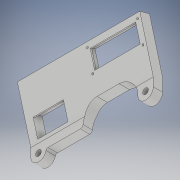
# Autodesk Inventor part: dash
Saved by Autodesk Inventor 2019 (Build 230136000, 136)
## iProperties
Created: 2019-09-21
Part Number: dash
Material: Generic
Document SubType Name: Modeling
Designer: steve
Density: 1 g/cm^3
Appearance: Default
Author: steve
Autodesk Inventor part; units mm, degrees
ref_plane "YZ Plane" through (0, 0, 0) normal (1, 0, 0) x (0, 1, 0)
ref_plane "XZ Plane" through (0, 0, 0) normal (0, 1, 0) x (-1, 0, 0)
ref_plane "XY Plane" through (0, 0, 0) normal (0, 0, 1) x (1, 0, 0)
sketch "Sketch1" plane through (0, 0, 0) normal (0, 1, 0) x (-1, 0, 0)
  line L0 (0, 0) -> (0, -18.7068)
  line L1 (0, -18.7068) -> (19.6073, -91.8823)
  line L2 (0, 0) -> (0, 11.24)
  line L3 (0, 11.24) -> (14, 11.24)
  line L4 (14, 11.24) -> (14, -13)
  line L5 (14, -13) -> (34.0962, -88)
  line L6 (34.0962, -88) -> (19.6073, -91.8823)
  dimension "d1" = 14
  dimension "d2" = 11.24
  dimension "d4" = 15
  dimension "d13" = 15
  dimension "d14" = 13
  dimension "d35" = 88
  constraints: 14 end point, 3 perpendicular, 2 vertical, 1 parallel
  measures "d1" distance of L2.end L3.end
  measures "d2" distance of L0.start L2.end
  measures "d4" angle of L0 L1
  measures "d13" distance of L5.end L1.end
  measures "d14" vertical distance of L4.end L0.start
  measures "d35" vertical distance of L5.end L0.start
extrude "Extrusion1" add sketch "Sketch1" along normal blind 183
sketch "Sketch2" plane through (-14, 0, -13) normal (-1, 0, 0) x (0, 0, 1)
  line L0 (0, 183) -> (24.24, 183) projected
  circle A0 centre (12.74, 171.5) radius 4.25
  circle A1 centre (12.74, 11.5) radius 4.25
  line L1 (24.24, 0) -> (24.24, 183) projected
  line L2 (0, 0) -> (24.24, 0) projected
  arc A2 (12.74, 0) -> (15.1193, 22.7512) centre (12.74, 11.5) ccw
  arc A3 (12.2608, 160.01) -> (12.74, 183) centre (12.74, 171.5) ccw
  line L3 (-13.26, 102.4155) -> (-13.26, 135.5313)
  arc A4 (12.2608, 160.01) -> (-13.26, 135.5313) centre (11.24, 135.5313) ccw
  circle A5 centre (20.1015, 118.5) radius 28 construction
  line L4 (12.74, 25.6863) -> (12.74, 74.0254)
  arc A6 (12.74, 25.6863) -> (15.1193, 22.7512) centre (15.74, 25.6863) ccw
  arc A7 (-13.26, 102.4155) -> (9.0909, 78.01) centre (11.24, 102.4155) ccw
  arc A8 (12.74, 74.0254) -> (9.0909, 78.01) centre (8.74, 74.0254) ccw
  line L5 (24.24, 0) -> (24.24, 183) projected
  line L6 (12.74, 0) -> (24.24, 0)
  line L7 (24.24, 11.5) -> (24.24, 171.5)
  line L8 (24.24, 183) -> (12.74, 183)
  line L9 (24.24, 11.5) -> (24.24, 0)
  line L10 (24.24, 171.5) -> (24.24, 183)
  point P0 (13, 0)
  point P1 (12.74, 23)
  point P2 (12.74, 77.9615)
  dimension "d17" = 160
  dimension "d18" = 183
  dimension "d19" = 11.5
  dimension "d20" = 11.5
  dimension "d21" = 11.5
  dimension "d22" = 26
  dimension "d23" = 56
  dimension "d24" = 53
  dimension "d25" = 3
  dimension "d26" = 0
  dimension "d27" = 24.5
  dimension "d28" = 4
  dimension "d30" = 82
  dimension "d31" = 8.5
  dimension "d32" = 4.1385
  constraints: 16 point on circle, 14 end point, 11 tangent, 9 centre point, 4 collinear, 4 point on line, 2 coincident, 2 equal radius, 2 vertical, 1 perpendicular
  measures "d17" distance of A0.centre A1.centre
  measures "d18" distance of L1.start L0.end
  measures "d19" distance from line of L2 A1.centre
  measures "d20" distance from line of L1 A1.centre
  measures "d21" distance from line of L1 A0.centre
  measures "d22" distance from line of A1.centre L3
  measures "d23" diameter of A5
  measures "d24" vertical distance of A0.centre A5.centre
  measures "d25" radius of A6
  measures "d26" distance from line of A1.centre L4
  measures "d27" radius of A4
  measures "d28" radius of A8
  measures "d30" vertical distance of A3.start A7.end
  measures "d31" diameter of A1
  measures "d32" distance from line of A5.centre L1
extrude "Extrusion2" cut sketch "Sketch2" along normal through all both and the other way through all
sketch "Sketch3" plane through (-34.0962, 0, -88) normal (-0.9659258, 0, 0.258819) x (0.258819, 0, 0.9659258)
  line L0 (46.9516, 11.5) -> (72.9516, 11.5)
  line L1 (72.9516, 11.5) -> (72.9516, 56.75)
  line L2 (72.9516, 56.75) -> (46.9516, 56.75)
  line L3 (46.9516, 56.75) -> (46.9516, 11.5)
  ellipse E0 centre (89.9516, 11.5) end of major axis (89.9516, 23) minor radius 11.1081 (89.9516, 0) -> (92.2498, 22.7512) ccw projected
  line L4 (8.9516, 106.5) -> (34.9516, 106.5)
  line L5 (34.9516, 106.5) -> (34.9516, 174.5)
  line L6 (34.9516, 174.5) -> (8.9516, 174.5)
  line L7 (8.9516, 174.5) -> (8.9516, 106.5)
  circle A0 centre (6.4516, 103) radius 1.4
  circle A1 centre (37.4516, 103) radius 1.4
  circle A2 centre (37.4516, 178) radius 1.4
  circle A3 centre (6.4516, 178) radius 1.4
  line L8 (6.4516, 103) -> (37.4516, 103) construction
  line L9 (37.4516, 103) -> (37.4516, 178) construction
  line L10 (37.4516, 178) -> (6.4516, 178) construction
  line L11 (6.4516, 178) -> (6.4516, 103) construction
  point P0 (93.8262, 0)
  dimension "d36" = 45.25
  dimension "d37" = 26
  dimension "d38" = 17
  dimension "d39" = 0
  dimension "d46" = 26
  dimension "d47" = 31
  dimension "d48" = 75
  dimension "d49" = 3.5
  dimension "d50" = 68
  dimension "d51" = 2.5
  dimension "d52" = 55
  dimension "d53" = 95
  dimension "d54" = 2.8
  constraints: 24 end point, 6 parallel, 4 centre point, 3 equal radius, 3 horizontal, 3 perpendicular, 2 coincident, 1 other
  measures "d36" distance of L2.end L0.start
  measures "d37" distance of L1.end L2.end
  measures "d38" distance from line of point (89.952, 11.5) L1
  measures "d39" distance from line of point (89.952, 11.5) L0
  measures "d46" distance of L4.start L4.end
  measures "d47" distance of L9.end L10.end
  measures "d48" distance of L10.end L8.start
  measures "d49" distance between parallel lines of L8 L4
  measures "d50" distance of L6.end L4.start
  measures "d51" distance between parallel lines of L11 L7
  measures "d52" horizontal distance of point (89.952, 11.5) L4.end
  measures "d53" vertical distance of point (89.952, 11.5) L4.end
  measures "d54" diameter of A0
extrude "top" cut sketch "Sketch3" against normal blind 183
sketch "Sketch4" plane through (-19.6073, 0, -91.8823) normal (0.9659258, 0, -0.258819) x (-0.258819, 0, -0.9659258)
  line L0 (-46.9516, 56.75) -> (-46.9516, 11.5) projected
  line L1 (-72.9516, 11.5) -> (-72.9516, 56.75) projected
  line L2 (-42.9516, 56.75) -> (-76.9516, 56.75)
  line L3 (-76.9516, 56.75) -> (-76.9516, 11.5)
  line L4 (-76.9516, 11.5) -> (-42.9516, 11.5)
  line L5 (-42.9516, 11.5) -> (-42.9516, 56.75)
  line L6 (-72.9516, 56.75) -> (-46.9516, 56.75) projected
  line L7 (-46.9516, 11.5) -> (-72.9516, 11.5) projected
  line L8 (-3.9516, 180.5) -> (-39.9516, 180.5)
  line L9 (-39.9516, 180.5) -> (-39.9516, 100.5)
  line L10 (-39.9516, 100.5) -> (-3.9516, 100.5)
  line L11 (-3.9516, 100.5) -> (-3.9516, 180.5)
  circle A0 centre (-6.4516, 103) radius 1.4 projected
  circle A1 centre (-6.4516, 178) radius 1.4 projected
  circle A2 centre (-37.4516, 178) radius 1.4 projected
  point P0 (-93.8262, 0)
  dimension "d42" = 4
  dimension "d43" = 4
  dimension "d55" = 2.5
  dimension "d56" = 2.5
  dimension "d57" = 2.5
  dimension "d59" = 2.5
  constraints: 16 end point, 4 parallel, 2 collinear, 2 horizontal, 2 perpendicular
  measures "d42" distance between parallel lines of L0 L5
  measures "d43" distance between parallel lines of L3 L1
  measures "d55" distance from line of L11 A0.centre
  measures "d56" distance from line of A0.centre L10
  measures "d57" distance from line of A1.centre L8
  measures "d59" distance from line of L9 A2.centre
extrude "back" cut sketch "Sketch4" against normal blind 12.6 contours L2 L5 L4 L0 | L1 L4 L3 L2 | L11 L10 L9 L8
equation "\"d19\" = -0.5 * d17 + 0.5 * d18"
equation "\"d21\" = d20"
equation "\"d49\" = -0.5 * d50 + 0.5 * d48"
equation "\"d51\" = -0.5 * d46 + 0.5 * d47"
equation "\"d43\" = d42"
equation "\"d56\" = d55"
equation "\"d57\" = d55"
equation "\"d59\" = d55"
body "Solid1"
